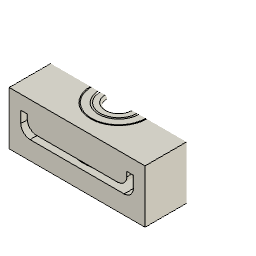
Scheinwerferhalterung v18 (Autodesk Fusion 360 design; units mm, degrees)
Autodesk Fusion 360 part; units mm, degrees
note: some values were not read from the file. Chosen so that the rebuilt part matches the saved one: which bodies a step acts on; which face or edge a step refers to. Set by a fixed rule: which sketch regions a step uses.
sketch "Skizze17" plane through (0, 0, 0) normal (0, 0, 1) x (1, 0, 0)
  line L0 (8, -8) -> (-8, -8)
  line L1 (-8, -8) -> (-8, 8)
  line L2 (-8, 8) -> (8, 8)
  line L3 (8, 8) -> (8, -8)
  line L4 (8, -8) -> (-8, 8) construction
  line L5 (-8, -8) -> (8, 8) construction
  dimension "d86" = 16
  dimension "d87" = 16
  constraint horizontal L0
  constraint perpendicular L0 L1
  constraint parallel L0 L2
  constraint parallel L1 L3
  constraint coincident L4 origin
  constraint coincident L5 origin
  measures "d86" distance of L1.end L2.end
  measures "d87" distance of L0.end L1.end
extrude "Extrusion10" add sketch "Skizze17" along normal blind 6 makes body 1
ref_plane "Arbeitsebene11" through (0, 0, 3) normal (0, 0, 1) x (1, 0, 0)
sketch "Skizze18" plane through (0, 0, 3) normal (0, 0, 1) x (1, 0, 0)
sphere "Grundkörper Kugel3" add diameter 10 placed x (1, 0, 0) y (0, 1, 0) z (0, 0, 1) at (0, 0, 3) separate body makes body 2
split "Teilen4" by bodies 2 bodies 1 makes body 3 at (0.0996, -6.6629, 0)
move_face "Flächen versetzen1" offset -0.3 1 faces at (3.714, -3.3441, 3.1532) on bodies 3
extrude "Extrusion11" cut sketch "Skizze17" along normal blind 3.163 from surface at 6 bodies 2
extrude "Extrusion12" cut sketch "Skizze17" against normal blind 10 bodies 2
sphere "Grundkörper Kugel4" cut diameter 7 placed x (1, 0, 0) y (0, 1, 0) z (0, 0, 1) at (0, 0, 3) bodies 2
extrude "Extrusion13" cut sketch "Skizze17" along normal blind 0.4 bodies 2
sketch "Skizze21" plane through (0, 0, 0) normal (0, 0, 1) x (1, 0, 0)
  line L0 (-0.75, -10) -> (0.75, -10)
  line L1 (0.75, -10) -> (0.75, 10)
  line L2 (0.75, 10) -> (-0.75, 10)
  line L3 (-0.75, 10) -> (-0.75, -10)
  line L4 (-0.75, -10) -> (0.75, 10) construction
  line L5 (0.75, -10) -> (-0.75, 10) construction
  line L6 (-10, -0.75) -> (10, -0.75)
  line L7 (10, -0.75) -> (10, 0.75)
  line L8 (10, 0.75) -> (-10, 0.75)
  line L9 (-10, 0.75) -> (-10, -0.75)
  line L10 (-10, -0.75) -> (10, 0.75) construction
  line L11 (10, -0.75) -> (-10, 0.75) construction
  dimension "d101" = 1.5
  dimension "d102" = 20
  dimension "d103" = 20
  dimension "d104" = 1.5
  constraint horizontal L0
  constraint perpendicular L0 L1
  constraint parallel L0 L2
  constraint parallel L1 L3
  constraint coincident L4 origin
  constraint coincident L5 origin
  constraint horizontal L6
  constraint perpendicular L6 L7
  constraint parallel L6 L8
  constraint parallel L7 L9
  constraint coincident L10 origin
  constraint coincident L11 origin
  measures "d101" distance of L1.end L2.end
  measures "d102" distance of L0.end L1.end
  measures "d103" distance of L7.end L8.end
  measures "d104" distance of L6.end L7.end
extrude "Extrusion14" cut sketch "Skizze21" along normal blind 5 contours L0 L1 L3 L6 | L3 L6 L8 L9 | L1 L6 L7 L8 | L1 L2 L3 L8 bodies 2
fillet "Abrundung5" radius 0.75 8 edges at (0.75, 3.6467, 5) (-0.75, 3.6467, 5) (3.6467, -0.75, 5) (3.6467, 0.75, 5) (-0.75, -3.6467, 5) (0.75, -3.6467, 5) (-3.6467, 0.75, 5) (-3.6467, -0.75, 5) on bodies 2
fillet "untere innere oeffnung" radius 0.7 4 edges at (-1.6568, -1.6568, 0.4) (1.6568, -1.6568, 0.4) (1.6568, 1.6568, 0.4) (-1.6568, 1.6568, 0.4) on bodies 2
fillet "Abrundung7" radius 0.4 1 edges at (-0.6519, -1.6808, 6) on bodies 2
sketch "Skizze27" plane through (0, 0, 6) normal (0, 0, 1) x (-1, 0, 0)
  circle A0 centre (0, 0) radius 4.3692
  line L0 (-8, -8) -> (8, -8)
  line L1 (8, -8) -> (8, 8)
  line L2 (8, 8) -> (-8, 8)
  line L3 (-8, 8) -> (-8, -8)
  circle A1 centre (0, 0) radius 5.8692
  dimension "d136" = 1.5
extrude "Extrusion19" add sketch "Skizze27" against normal blind 11.451 draft 15 separate body contours A1 makes body 4
split "Teilen5" by bodies 4 bodies 3 makes body 5 at (-0.1462, -7.2843, 6)
sketch "Skizze25" plane through (0, 0, 0) normal (0, 1, 0) x (1, 0, 0)
  line L0 (0, 0) -> (0, 1.5) construction
  line L1 (-10.15, 1.5) -> (10.15, 1.5)
  line L2 (-12.15, -0.5) -> (-12.15, -3)
  line L3 (-12.15, -3) -> (-10.75, -3)
  line L4 (-10.75, -3) -> (-10.75, -2)
  line L5 (0, 0) -> (-8.75, 0)
  line L6 (12.15, -0.5) -> (12.15, -3)
  line L7 (12.15, -3) -> (10.75, -3)
  line L8 (10.75, -3) -> (10.7501, -2.0002)
  line L9 (0, 0) -> (8.7501, 0)
  arc A0 (12.15, -0.5) -> (10.15, 1.5) centre (10.15, -0.5) ccw
  arc A1 (10.7501, -2.0002) -> (8.7501, 0) centre (8.7501, -2) ccw
  arc A2 (-10.15, 1.5) -> (-12.15, -0.5) centre (-10.15, -0.5) ccw
  arc A3 (-8.75, 0) -> (-10.75, -2) centre (-8.75, -2) ccw
  line L10 (14.6757, 5.4987) -> (-14.6757, 5.4987)
  line L11 (-14.6757, 5.4987) -> (-14.6757, -6)
  line L12 (-14.6757, -6) -> (14.6757, -6)
  line L13 (14.6757, -6) -> (14.6757, 5.4987)
  line L14 (-8, 0) -> (8, 0)
  line L15 (8, 0) -> (8, -6)
  line L16 (8, -6) -> (-8, -6)
  line L17 (-8, -6) -> (-8, 0)
  point P0 (-12.15, 1.5)
  point P1 (12.15, 1.5)
  dimension "d113" = 1.5
  dimension "d117" = 2
  dimension "d118" = 4.5
  dimension "d120" = 24.3
  dimension "d121" = 1.4
  constraint vertical L0
  constraint coincident L0.start L5.start
  constraint horizontal L1
  constraint vertical L2
  constraint perpendicular L2 L3
  constraint vertical L4
  constraint symmetric L0 L2.end L6.end
  constraint symmetric L0 L3.end L7.end
  constraint symmetric L0 L5.start L9.start
  constraint coincident L0.end L1
  constraint coincident P1 L1
  constraint tangent L1 A0
  constraint tangent L6 A0
  constraint tangent L9 A1
  constraint tangent L8 A1
  constraint equal A0 A1
  constraint coincident P0 L1
  constraint coincident P0 L2
  constraint tangent L1 A2
  constraint tangent L2 A2
  constraint equal A0 A2
  constraint tangent L4 A3
  constraint tangent L5 A3
  constraint equal A0 A3
  constraint horizontal L5
  constraint horizontal L9
  constraint horizontal L10
  constraint vertical L11
  constraint horizontal L12
  constraint vertical L13
  constraint midpoint L12 L16
  measures "d113" distance of L0.start L0.end
  measures "d117" radius of A0
  measures "d118" distance of L1 L3
  measures "d120" distance of L2 L6
  measures "d121" distance of L2 L4
extrude "Extrusion15" add sketch "Skizze25" along normal mid plane 16 contours L1 L2 L3 L4 L5 L6 L7 L8 L9 A0 A1 A2 A3 L10 L11 L12 L13 L15 L17 bodies 5
move_face "Flächen versetzen2" offset -0.2 1 faces at (-6.4146, 3.0891, 1.3333) on bodies 5
sketch "Skizze28" plane through (0, 0, -5.4987) normal (0, 0, -1) x (1, 0, 0)
  line L0 (-14.6757, 8) -> (-14.6757, -8)
  line L1 (-14.6757, -8) -> (14.6757, -8)
  line L2 (14.6757, -8) -> (14.6757, 8)
  line L3 (14.6757, 8) -> (-14.6757, 8)
  circle A0 centre (0, 0) radius 7.684
  line L4 (-8.75, -8) -> (8.7501, -8)
  line L5 (8.7501, -8) -> (8.7501, 8)
  line L6 (8.7501, 8) -> (-8.75, 8)
  line L7 (-8.75, 8) -> (-8.75, -8)
extrude "Extrusion20" cut sketch "Skizze28" against normal up to surface (3.9987 mm away) contours A0 bodies 5
extrude "Extrusion21" add 1 faces at (3.3833, -8, -4.1658) along direction (0, -1, 0) blind 1 on bodies 5 bodies 5
sketch "Skizze29" plane through (0, 8, 0) normal (0, 1, 0) x (-1, 0, 0)
  line L0 (-8.7501, 0) -> (8.75, 0)
  arc A0 (8.75, 0) -> (10.75, 2) centre (8.75, 2) ccw
  line L1 (10.75, 2) -> (10.75, 3)
  line L2 (10.75, 3) -> (12.15, 3)
  line L3 (12.15, 3) -> (12.15, 0.5)
  arc A1 (10.15, -1.5) -> (12.15, 0.5) centre (10.15, 0.5) ccw
  line L4 (10.15, -1.5) -> (-10.15, -1.5)
  arc A2 (-12.15, 0.5) -> (-10.15, -1.5) centre (-10.15, 0.5) ccw
  line L5 (-12.15, 0.5) -> (-12.15, 3)
  line L6 (-12.15, 3) -> (-10.75, 3)
  line L7 (-10.75, 3) -> (-10.7501, 2.0002)
  arc A3 (-10.7501, 2.0002) -> (-8.7501, 0) centre (-8.7501, 2) ccw
  line L8 (14.6757, 6) -> (-14.6757, 6)
  line L9 (-14.6757, 6) -> (-14.6757, -5.4987)
  line L10 (-14.6757, -5.4987) -> (14.6757, -5.4987)
  line L11 (14.6757, -5.4987) -> (14.6757, 6)
  line L12 (-12.15, 3) -> (-10.7497, 3)
  line L13 (-10.7497, 3) -> (-10.7497, 6)
  line L14 (-10.7497, 6) -> (-12.15, 6)
  line L15 (-12.15, 6) -> (-12.15, 3)
  line L16 (10.75, 3) -> (12.15, 3)
  line L17 (12.15, 3) -> (12.15, 6)
  line L18 (12.15, 6) -> (10.75, 6)
  line L19 (10.75, 6) -> (10.75, 3)
  line L20 (2, -1.5) -> (-2, -1.5)
  line L21 (-2, -1.5) -> (-2, -4)
  line L22 (-2, -4) -> (2, -4)
  line L23 (2, -4) -> (2, -1.5)
  dimension "d148" = 4
  dimension "d149" = 2.5
  constraint horizontal L12
  constraint vertical L13
  constraint horizontal L14
  constraint vertical L15
  constraint coincident L8 L13.end
  constraint coincident L5.end L6.start
  constraint horizontal L16
  constraint vertical L17
  constraint horizontal L18
  constraint vertical L19
  constraint coincident L8 L17.end
  constraint coincident L1.end L2.start
  constraint horizontal L20
  constraint vertical L21
  constraint horizontal L22
  constraint vertical L23
  constraint midpoint L4 L20
  measures "d148" distance of L20.start L20.end
  measures "d149" distance of L20.start L22.end
extrude "Extrusion22" add sketch "Skizze29" along normal blind 5 contours L0 A0 L1 L7 A3 L8 L13 L19 | L3 A1 L4 A2 L5 L8 L9 L10 L11 L15 L17 L21 L22 L23 bodies 5
extrude "Extrusion23" cut sketch "Skizze29" against normal blind 3 contours L6 L8 L12 L13 L14 L15 | L2 L8 L16 L17 L18 L19 bodies 5
hidden bodies 1 4
equation "d88 = 6 mm"
equation "d90 = d88 / 2"
equation "d91 = 10 mm"
equation "d104 = d101"
equation "d105 = d91 * 0,5"
equation "d108 = d101 / 2"
named bodies: "aussen", "innen", "konische Fassung", "Teilungskoerper", "Body"
